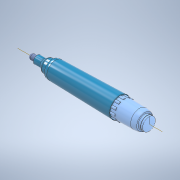
# Autodesk Inventor part: marcador
Saved by Autodesk Inventor 2021.5 (Build 255421000, 421)
## iProperties
Created: 2024-11-16
Part Number: marcador
Material: Marcador Plastico
Document SubType Name: Modeling
Designer: Joho_
Density: 0.701 g/cm^3
Appearance: Genérico
Mass: 23.0179 g
Surface Area: 74.4274 cm^2
Volume: 32.8359 cm^3
Author: Joho_
Autodesk Inventor part; units mm, degrees
ref_plane "YZ Plane" through (0, 0, 0) normal (1, 0, 0) x (0, 1, 0)
ref_plane "XZ Plane" through (0, 0, 0) normal (0, 1, 0) x (-1, 0, 0)
ref_plane "XY Plane" through (0, 0, 0) normal (0, 0, 1) x (1, 0, 0)
sketch "Boceto1" plane through (0, 0, 0) normal (0, 0, 1) x (1, 0, 0)
  line L0 (-103.5851, 10.8479) -> (31.8816, 10.8479) construction
  line L1 (31.8816, 10.8479) -> (31.8816, -10.8479) construction
  line L2 (31.8816, -10.8479) -> (-103.5851, -10.8479) construction
  line L3 (-103.5851, -10.8479) -> (-103.5851, 10.8479) construction
  line L4 (0, 0) -> (-71.5, 0)
  line L5 (0, 10.9) -> (0, 0)
  line L6 (-68.2708, 0) -> (0, 0)
  line L7 (0, 10.9) -> (-68.1013, 9.2541)
  line L8 (-71.5, 0) -> (-56.9274, 0) construction
  line L9 (-71.5, 0) -> (-71.5, 8.5)
  line L10 (-71.5, 0) -> (-68, 0)
  line L11 (-68, 0) -> (-68, 9.2565)
  arc A0 (-68, 9.2565) -> (-71.5, 8.5) centre (-67.8264, -0.0207) ccw
  line L12 (-68, 9.2565) -> (0, 10.9)
  line L13 (0, 0) -> (26.5, 0)
  line L14 (26.5, 0) -> (26.5, 7)
  line L15 (0, 0) -> (0, 9.9)
  line L16 (0, 0) -> (21, 0)
  line L17 (21, 0) -> (21, 9.5)
  line L18 (21, 9.5) -> (0, 9.9)
  line L19 (26.5, 0) -> (26.5, 8.5)
  arc A1 (26.5, 8.5) -> (21, 9.5) centre (21.692, -2.3188) ccw
  line L20 (26.5, 0) -> (29, 0)
  line L21 (29, 0) -> (29, 7)
  line L22 (29, 7) -> (26.5, 7)
  line L23 (29, 0) -> (29, 6.75)
  line L24 (29, 6.75) -> (31, 6.75)
  line L25 (31.8816, 6.75) -> (31.8816, 0)
  line L26 (31.8816, 0) -> (29, 0)
  line L27 (29, 0) -> (29, 6.75)
  line L28 (29, 6.75) -> (31, 6.75)
  line L29 (29, 0) -> (31, 0)
  ellipse E0 centre (31, 0) end of major axis (31, 6.75) minor radius 0.8816 (30.1184, 0) -> (31, 6.75) ccw
  ellipse E1 centre (31, 0) end of major axis (31, 6.75) minor radius 0.8816 (31, 6.75) -> (30.1184, 0) ccw
  line L30 (31, 6.75) -> (31.8816, 6.75)
  line L31 (-71.5, 0) -> (-71.5, 7.25)
  line L32 (-71.5, 0) -> (-67, 0)
  line L33 (-71.5, 0) -> (-76, 0)
  line L34 (-76, 0) -> (-76, 6.75)
  line L35 (-76, 6.75) -> (-71.5, 7.25)
  line L36 (-76, 0) -> (-77, 0)
  line L37 (-77, 0) -> (-77, 6.5)
  line L38 (-77, 6.5) -> (-76, 6.75)
  line L39 (-77, 0) -> (-80.5, 0)
  line L40 (-80.5, 0) -> (-80.5, 4.15)
  line L41 (-80.5, 4.15) -> (-77, 6.5)
  line L42 (-80.5, 0) -> (-87.5, 0)
  line L43 (-87.5, 0) -> (-87.5, 4.15)
  line L44 (-87.5, 4.15) -> (-80.5, 4.15)
  line L45 (-80.5, 4.15) -> (-80.5, 0)
  line L46 (-87.5, 0) -> (-95, 0)
  line L47 (-95, 0) -> (-95, 0)
  line L48 (-92.25, 2.75) -> (-87.5, 2.75)
  line L49 (-87.5, 2.75) -> (-87.5, 0)
  arc A2 (-92.25, 2.75) -> (-95, 0) centre (-92.25, 0) ccw
  point P0 (67.7333, -10.8479)
  point P1 (103.6012, -10.8479)
  point P2 (35.8517, 0)
  point P3 (7, 16)
  point P4 (-95, 2.75)
  dimension "d16" = 71.5
  dimension "d27" = 8.5
  dimension "d29" = 3.5
  dimension "d42" = 26.5
  dimension "d43" = 7
  dimension "d45" = 9.9
  dimension "d46" = 21
  dimension "d47" = 9.5
  dimension "d48" = 8.5
  dimension "d55" = 2.5
  dimension "d56" = 6.75
  dimension "d59" = 2
  dimension "d60" = 2
  dimension "d63" = 7.25
  dimension "d64" = 4.5
  dimension "d65" = 4.5
  dimension "d66" = 6.75
  dimension "d67" = 1
  dimension "d68" = 6.5
  dimension "d69" = 3.5
  dimension "d70" = 4.15
  dimension "d71" = 7
  dimension "d72" = 7.5
  dimension "d73" = 2.75
  dimension "d74" = 2.75
  constraints: 94 end point, 12 horizontal, 12 point on line, 10 perpendicular, 7 parallel, 7 point on circle, 4 coincident, 3 centre point, 3 vertical, 2 tangent, 1 collinear, 1 midpoint, 11 other
  measures "d16" distance of L4.start L4.end
  measures "d27" distance of L4.end L9.end
  measures "d29" distance of L4.end L10.end
  measures "d42" distance of L4.start L13.end
  measures "d43" distance of L13.end L14.end
  measures "d45" distance of L4.start L15.end
  measures "d46" distance of L4.start L16.end
  measures "d47" distance of L16.end L17.end
  measures "d48" distance of L13.end L19.end
  measures "d55" distance of L13.end L20.end
  measures "d56" distance of L20.end L23.end
  measures "d59" distance of L23.end L24.end
  measures "d60" distance of L26.end L29.end
  measures "d63" distance of L4.end L31.end
  measures "d64" distance of L4.end L32.end
  measures "d65" distance of L4.end L33.end
  measures "d66" distance of L33.end L34.end
  measures "d67" distance of L33.end L36.end
  measures "d68" distance of L36.end L37.end
  measures "d69" distance of L36.end L39.end
  measures "d70" distance of L39.end L40.end
  measures "d71" distance of L43.end L44.end
  measures "d72" distance of point (-95, 2.75) L48.end
  measures "d73" distance of L46.end point (-95, 2.75)
  measures "d74" radius of A2
revolve "Revolución1" add sketch "Boceto1" angle 360 about axis through (0, 0, 0) along (-1, 0, 0) contours L4 L11 L7 L5 | L4 L9 A0 L7 L11
sketch "Boceto2" plane through (0, 0, 0) normal (1, 0, 0) x (0, 0, -1)
  arc A0 (1.1877, 9.8285) -> (-1.1877, 9.8285) centre (0, 0) ccw
  line L0 (0, 9.9) -> (0, 10.6)
  line L1 (0, 10.6) -> (0, 9.3)
  arc A1 (1.1877, 9.8285) -> (-1.1877, 9.8285) centre (0, 9.3) ccw
  arc A2 (-1.1877, 9.8285) -> (1.1877, 9.8285) centre (0, 0) ccw
  circle A3 centre (0, 9.3) radius 1.3
  point P0 (-1.1877, 9.8285)
  point P1 (1.1877, 9.8285)
  dimension "d38" = 19.8
  dimension "d39" = 0.7
  dimension "d40" = 1.3
  constraints: 8 point on circle, 4 centre point, 4 end point, 3 coincident, 2 vertical, 1 concentric
  measures "d38" diameter of A0
  measures "d39" distance of L0.start L0.end
  measures "d40" distance of L0.end L1.end
revolve "Revolución2" add sketch "Boceto1" angle 360 about axis through (0, 0, 0) along (1, 0, 0) contours L5 L18 L17 L13 | L17 A1 L19 L14 L13
extrude "Extrusión1" add sketch "Boceto2" along normal blind 5 contours A3 A0 | A0 L0 A1 | A0 A1 L0
pattern_circular "Patrón circular1" count 12 over 360 about axis through (-10, 0, 0) along (1, 0, 0) of "Extrusión1"
revolve "Revolución3" add sketch "Boceto1" angle 360 about axis through (26.5, 0, 0) along (1, 0, 0) contours L14 L22 L21 L20 | L21 L24 E1 L26 | E1 E0 L26
revolve "Revolución4" add sketch "Boceto1" angle 360 about axis through (-80.5, 0, 0) along (-1, 0, 0) contours L33 L34 L35 L9 | L36 L37 L38 L34 | L39 L40 L41 L37 | L42 L43 L44 L40
revolve "Revolución5" add sketch "Boceto1" angle 360 about axis through (-87.5, 0, 0) along (-1, 0, 0) contours L46 A2 L48 L43
